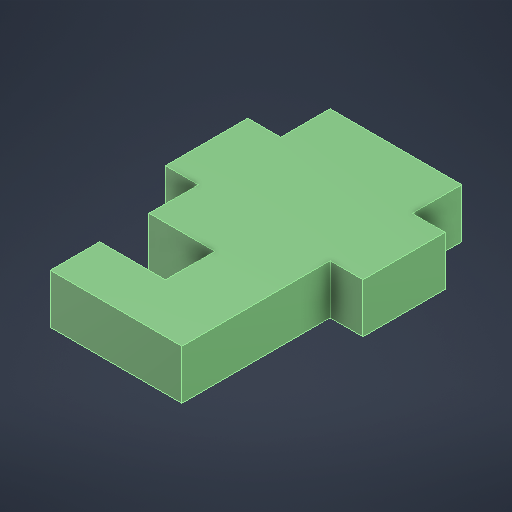
# Autodesk Inventor part: plug
Saved by Autodesk Inventor 2025.3 (Build 293356030, 356C)
## iProperties
Created: 2025-09-04
Part Number: plug
Material: 木材 (楓木)
Document SubType Name: Modeling
Designer: 陳泓任
Density: 0.67 g/cm^3
Appearance: 平滑 - 深森林綠
Author: 陳泓任
Autodesk Inventor part; units mm, degrees
ref_plane "YZ Plane" through (0, 0, 0) normal (1, 0, 0) x (0, 1, 0)
ref_plane "XZ Plane" through (0, 0, 0) normal (0, 1, 0) x (-1, 0, 0)
ref_plane "XY Plane" through (0, 0, 0) normal (0, 0, 1) x (1, 0, 0)
sketch "草圖1" plane through (0, 0, 0) normal (0, 1, 0) x (-1, 0, 0)
  line L0 (4, 11.5) -> (-4, 11.5)
  line L1 (-4, -5.5) -> (4, -5.5)
  line L2 (-6, 2.5) -> (-6, -2.5)
  line L3 (6, -2.5) -> (6, 2.5)
  line L4 (6, 2.5) -> (4, 2.5)
  line L5 (-4, 2.5) -> (-6, 2.5)
  line L6 (4, -5.5) -> (4, -2.5)
  line L7 (-6, -2.5) -> (-4, -2.5)
  line L8 (4, -2.5) -> (6, -2.5)
  line L9 (-4, 11.5) -> (-4, 2.5)
  line L10 (-4, -2.5) -> (-4, -5.5)
  line L11 (0, 14.8546) -> (0, -17.157)
  line L12 (13.4413, 0) -> (-16.1444, 0)
  line L13 (4, 5.5) -> (0, 5.5)
  line L14 (0, 5.5) -> (0, 8.5)
  line L15 (0, 8.5) -> (4, 8.5)
  line L16 (4, 2.5) -> (4, 5.5)
  line L17 (4, 8.5) -> (4, 11.5)
  point P0 (0, 0)
  point P1 (-6, 0)
  point P2 (6, 0)
  dimension "d0" = 8
  dimension "d3" = 5
  dimension "d5" = 12
  dimension "d8" = 3
  dimension "d9" = 9
  dimension "d10" = 3
  dimension "d11" = 3
  constraints: 36 end point, 13 parallel, 6 perpendicular, 4 collinear, 4 horizontal, 4 point on line, 2 midpoint, 1 vertical, 3 other
  measures "d0" distance of L0.start L0.end
  measures "d3" distance of L2.start L2.end
  measures "d5" distance between parallel lines of L2 L3
  measures "d8" distance of L7.end L1.start
  measures "d9" distance of L0.end L5.start
  measures "d10" distance of L4.end L13.start
  measures "d11" distance between parallel lines of L15 L13
extrude "擠出1" add sketch "草圖1" along normal blind 3
